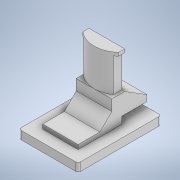
# Autodesk Inventor part: stopper
Saved by Autodesk Inventor 2021.1 (Build 251245010, 245A)
## iProperties
Created: 2021-08-22
Part Number: stopper
Material: Типовые
Document SubType Name: Modeling
Designer: User
Density: 1 g/cm^3
Appearance: По умолчанию
Author: User
Autodesk Inventor part; units mm, degrees
ref_plane "YZ Plane" through (0, 0, 0) normal (1, 0, 0) x (0, 1, 0)
ref_plane "XZ Plane" through (0, 0, 0) normal (0, 1, 0) x (-1, 0, 0)
sketch "Эскиз1" plane through (0, 0, 0) normal (0, 1, 0) x (-1, 0, 0)
  line L0 (-7.5, 14.5) -> (7.5, 14.5)
  line L1 (7.5, 14.5) -> (7.5, -14.5)
  line L2 (7.5, -14.5) -> (-7.5, -14.5)
  line L3 (-7.5, -14.5) -> (-7.5, 14.5)
  line L4 (-7.5, 14.5) -> (7.5, -14.5) construction
  line L5 (7.5, 14.5) -> (-7.5, -14.5) construction
  point P0 (0, 0)
  dimension "d0" = 15
  dimension "d1" = 29
  constraints: 12 end point, 2 midpoint, 2 parallel, 1 horizontal, 1 perpendicular
  measures "d0" distance of L1.end L2.end
  measures "d1" distance of L0.end L1.end
extrude "Выдавливание1" add sketch "Эскиз1" along normal blind 27
sketch "Эскиз2" plane through (0, 0, 0) normal (0, -1, 0) x (1, 0, 0)
  line L0 (12.5, 19.5) -> (-12.5, 19.5)
  line L1 (-12.5, 19.5) -> (-12.5, -15.5)
  line L2 (-12.5, -15.5) -> (12.5, -15.5)
  line L3 (12.5, -15.5) -> (12.5, 19.5)
  line L4 (7.5, 14.5) -> (7.5, -14.5) projected
  line L5 (-7.5, 14.5) -> (7.5, 14.5) projected
  point P0 (0, 0)
  dimension "d4" = 25
  dimension "d5" = 35
  dimension "d6" = 5
  dimension "d7" = 5
  constraints: 8 end point, 2 parallel, 1 horizontal, 1 perpendicular
  measures "d4" distance of L2.end L1.end
  measures "d5" distance of L1.end L0.end
  measures "d6" distance between parallel lines of L3 L4
  measures "d7" distance between parallel lines of L0 L5
extrude "Выдавливание2" add sketch "Эскиз2" along normal blind 3.5
fillet "Сопряжение1" radius 1 1 edges at (-12.5, -1.75, 19.5)
fillet "Сопряжение2" radius 1 2 edges at (12.5, -1.75, 19.5) (12.5, -1.75, -15.5)
fillet "Сопряжение3" radius 1 1 edges at (-12.5, -1.75, -15.5)
sketch "Эскиз3" plane through (7.5, 27, 14.5) normal (1, 0, 0) x (0, 0, -1)
  line L0 (14.2, 0) -> (14.2, -20.2)
  line L1 (0, -27) -> (0, 0) projected
  line L2 (0, 0) -> (29, 0) projected
  line L3 (29, -27) -> (-4, -27) projected
  line L4 (-4, -27) -> (29, -27) projected
  line L5 (18.4, -27) -> (18.4, -24)
  line L6 (18.4, -24) -> (29, -24)
  line L7 (29, -27) -> (29, 0) projected
  line L8 (29, 0) -> (0, 0) projected
  line L9 (19.6, 0) -> (19.6, -15.6)
  line L10 (19.6, -15.6) -> (29, -21.4)
  line L11 (0, -25.2) -> (9.2, -25.2)
  line L12 (9.2, -25.2) -> (14.2, -20.2)
  point P0 (14.5, -27)
  dimension "d17" = 3
  dimension "d18" = 9.4
  dimension "d43" = 5
  constraints: 14 end point, 6 point on line, 3 perpendicular, 1 horizontal, 1 vertical
  measures "d17" distance between parallel lines of L3 L6
  measures "d18" distance between parallel lines of L9 L7
  measures "d43" distance from line of L0.end L11
extrude "Выдавливание3" cut sketch "Эскиз3" against normal blind 23 contours L0 L12 L11 L1 L2 | L2 L7 L10 L9 | L5 L6 L7 L3
sketch "Эскиз5" plane through (0, 27, 0) normal (0, 1, 0) x (1, 0, 0)
  line L0 (-7.5, 3.9) -> (-7.5, -14.5) projected
  line L1 (7.5, -14.5) -> (7.5, 3.9) projected
  arc A0 (-7.5, 2.5) -> (7.5, 2.5) centre (0, 11.1446) ccw
  line L2 (-7.5, -0.3) -> (7.5, -0.3) projected
  line L3 (7.5, 5.1) -> (-7.5, 5.1) projected
  point P0 (0, 0)
  point P1 (0, -0.3)
  dimension "d23" = 2.6
  dimension "d24" = 2.6
  constraints: 2 point on circle, 2 point on line, 1 centre point, 1 tangent
  measures "d23" distance from line of L3 A0.start
  measures "d24" distance of L3.start A0.end
extrude "Выдавливание4" cut sketch "Эскиз5" against normal blind 15.6
sketch "Эскиз6" plane through (7.5, 11.4, -5.1) normal (0, 0, -1) x (-1, 0, 0)
  line L0 (0, 0) -> (0, 15.6) projected
  line L1 (0, 15.6) -> (15, 15.6) projected
  line L2 (0, 14.2) -> (1.2, 14.2)
  line L3 (1.2, 14.2) -> (1.2, 0)
  line L4 (1.2, 0) -> (0, 0)
  line L5 (0, 0) -> (0, 14.2)
  line L6 (15, 0) -> (15, 15.6)
  line L7 (13.8, 14.2) -> (13.8, 0)
  line L8 (13.8, 0) -> (15, 0)
  line L9 (0, 14.2) -> (1.2, 14.2)
  line L10 (13.8, 14.2) -> (15.1024, 14.2)
  point P0 (7.5, -11.4)
  point P1 (15, 14.2)
  dimension "d28" = 1.2
  constraints: 18 end point, 3 horizontal, 2 parallel, 1 perpendicular, 1 point on line
  measures "d28" distance of L3.end L4.end
extrude "Выдавливание5" cut sketch "Эскиз6" against normal blind 16
sketch "Эскиз7" plane through (7.5, 3, -14.5) normal (0, -1, 0) x (1, 0, 0)
  line L0 (0, 0) -> (0, 9.4) projected
  line L1 (0, 4.5) -> (-15, 4.5)
  line L2 (-15, 0) -> (-15, 10.6) projected
  line L3 (0, 0) -> (-15, 0) projected
  point P0 (-7.5, 14.5)
  dimension "d36" = 4.5
  constraints: 2 end point, 2 point on line, 1 horizontal
  measures "d36" distance between parallel lines of L1 L3
ref_plane "РабПлоскость1" through (-7.5, 3, -10) normal (0, 0, -1) x (-1, 0, 0)
sketch "Эскиз8" plane through (-7.5, 3, -10) normal (0, 0, -1) x (-1, 0, 0)
  line L0 (-15, 0) -> (0, 0) projected
  arc A0 (-7.5, -1) -> (-6, 0) centre (-7.5, 0.625) ccw
  line L1 (-15, 0) -> (0, 0) projected
  line L2 (-7.5, 0) -> (-7.5, -1.5688)
  point P0 (-7.5, -3)
  point P1 (-9, 0)
  constraints: 2 end point, 2 point on circle, 1 centre point, 1 midpoint, 1 point on line, 1 vertical
revolve "Вращение2" add sketch "Эскиз8" angle 360 about axis through (0, 3, -10) along (0, -1, 0)
